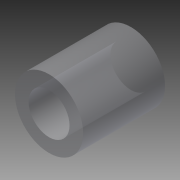
# Autodesk Inventor part: Climber Polycarbonate Spacer
Saved by Autodesk Inventor 2014 SP1 (Build 180222100, 222)
## iProperties
Created: 2013-10-27
Part Number: Climber Polycarbonate Spacer
Material: Polycarbonate, Clear
Document SubType Name: Modeling
Designer: Moses
Mass: 2.89583 g
Surface Area: 17.7348 cm^2
Volume: 2.41319 cm^3
Density: 1.2 g/cm^3
Appearance: Polycarbonate - Clear
Author: Moses
Autodesk Inventor part; units mm, degrees
ref_plane "YZ Plane" through (0, 0, 0) normal (1, 0, 0) x (0, 1, 0)
ref_plane "XZ Plane" through (0, 0, 0) normal (0, 1, 0) x (-1, 0, 0)
ref_plane "XY Plane" through (0, 0, 0) normal (0, 0, 1) x (1, 0, 0)
sketch "Sketch1" plane through (0, 0, 0) normal (0, 0, 1) x (1, 0, 0)
  circle A0 centre (0, 0) radius 4.7625
  circle A1 centre (0, 0) radius 7.9375
  dimension "d0" = 9.525
  dimension "d1" = 15.875
  constraints: 2 centre point, 2 coincident
  measures "d0" diameter of A0
  measures "d1" diameter of A1
extrude "Extrusion1" add sketch "Sketch1" along normal blind 19.05
body "Solid1"
